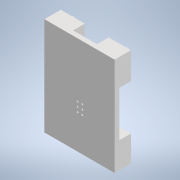
# Autodesk Inventor part: Soldering_Jig_Swerve
Saved by Autodesk Inventor 2022 (Build 260153000, 153)
## iProperties
Created: 2024-02-02
Part Number: Soldering_Jig_Swerve
Material: Generic
Document SubType Name: Modeling
Designer: Paul
Density: 1 g/cm^3
Appearance: Default
Author: Paul
Autodesk Inventor part; units mm, degrees
ref_plane "YZ Plane" through (0, 0, 0) normal (1, 0, 0) x (0, 1, 0)
ref_plane "XZ Plane" through (0, 0, 0) normal (0, 1, 0) x (-1, 0, 0)
ref_plane "XY Plane" through (0, 0, 0) normal (0, 0, 1) x (1, 0, 0)
sketch "Sketch1" plane through (0, 0, 0) normal (0, 0, 1) x (1, 0, 0)
  line L0 (-22.948, 8.421) -> (-22.948, -44.919) projected
  line L1 (-22.948, -44.919) -> (15.152, -44.919) projected
  line L2 (15.152, -44.919) -> (15.152, 8.421) projected
  line L3 (15.152, 8.421) -> (-22.948, 8.421) projected
  circle A0 centre (10.834, 4.103) radius 2.286 projected
  circle A1 centre (-18.63, 4.103) radius 2.286 projected
  circle A2 centre (-18.63, -40.601) radius 2.286 projected
  circle A3 centre (10.834, -40.601) radius 2.286 projected
  point P0 (0, 0)
extrude "Extrusion1" add sketch "Sketch1" along normal blind 2.54 contours L3 L2 L1 L0 | A0 | A1 | A2 | A3
sketch "Sketch2" plane through (0, 0, 0) normal (0, 0, -1) x (-1, 0, 0)
  line L0 (22.948, 8.421) -> (22.948, -44.919) projected
  line L1 (10.492, -0.541) -> (22.948, -0.541)
  line L2 (22.948, -0.541) -> (22.948, -18.939)
  line L3 (22.948, -18.939) -> (10.492, -18.939)
  line L4 (10.492, -18.939) -> (10.492, -0.541)
  line L5 (22.948, -22.163) -> (10.492, -22.163)
  line L6 (10.492, -22.163) -> (10.492, -35.163)
  line L7 (10.492, -35.163) -> (22.948, -35.163)
  line L8 (22.948, -35.163) -> (22.948, -22.163)
  line L9 (22.948, -44.919) -> (-15.152, -44.919) projected
  line L10 (8.874, -44.919) -> (-4.126, -44.919)
  line L11 (-4.126, -44.919) -> (-4.126, -32.448)
  line L12 (-4.126, -32.448) -> (8.874, -32.448)
  line L13 (8.874, -32.448) -> (8.874, -44.919)
  line L14 (-15.152, -44.919) -> (-15.152, 8.421) projected
  line L15 (-15.152, -30.845) -> (-2.427, -30.845)
  line L16 (-2.427, -30.845) -> (-2.427, -6.129)
  line L17 (-2.427, -6.129) -> (-15.152, -6.129)
  line L18 (-15.152, -6.129) -> (-15.152, -30.845)
  line L19 (-15.152, 8.421) -> (22.948, 8.421) projected
  line L20 (9.89, 8.421) -> (-3.11, 8.421)
  line L21 (-3.11, 8.421) -> (-3.11, -4.05)
  line L22 (-3.11, -4.05) -> (9.89, -4.05)
  line L23 (9.89, -4.05) -> (9.89, 8.421)
  line L24 (8.374, -32.948) -> (8.374, -44.198) projected
  line L25 (-3.626, -44.198) -> (-3.626, -32.948) projected
  line L26 (-1.876, -32.948) -> (-3.426, -32.948) projected
  line L27 (-2.927, -30.145) -> (-2.927, -28.595) projected
  line L28 (-2.927, -30.345) -> (-14.177, -30.345) projected
  line L29 (-2.927, -14.629) -> (-14.177, -14.629) projected
  line L30 (-14.177, -18.345) -> (-2.927, -18.345) projected
  line L31 (-14.177, -6.629) -> (-2.927, -6.629) projected
  line L32 (-2.41, -3.55) -> (-0.86, -3.55) projected
  line L33 (-2.61, -3.55) -> (-2.61, 7.7) projected
  line L34 (9.39, 7.7) -> (9.39, -3.55) projected
  line L35 (10.992, -1.041) -> (22.242, -1.041) projected
  line L36 (10.992, -1.241) -> (10.992, -2.791) projected
  line L37 (22.242, -9.041) -> (10.992, -9.041) projected
  line L38 (10.992, -10.439) -> (22.242, -10.439) projected
  line L39 (10.992, -10.639) -> (10.992, -12.189) projected
  line L40 (22.242, -18.439) -> (10.992, -18.439) projected
  line L41 (10.992, -22.663) -> (22.242, -22.663) projected
  line L42 (22.242, -34.663) -> (10.992, -34.663) projected
  line L43 (10.992, -32.913) -> (10.992, -34.463) projected
  point P0 (0, 0)
  dimension "d2" = 0.5
  dimension "d3" = 0.5
  dimension "d4" = 0.5
  dimension "d5" = 0.5
  dimension "d6" = 0.5
  dimension "d7" = 0.5
  dimension "d8" = 0.5
  dimension "d9" = 0.5
  dimension "d10" = 0.5
  dimension "d11" = 0.5
  dimension "d12" = 0.5
  dimension "d13" = 0.5
  dimension "d14" = 0.5
  dimension "d15" = 0.5
  constraints: 40 end point, 10 parallel, 6 point on line, 5 horizontal, 5 perpendicular
  measures "d2" distance between parallel lines of L6 L43
  measures "d3" distance between parallel lines of L42 L7
  measures "d4" distance between parallel lines of L5 L41
  measures "d5" distance between parallel lines of L40 L3
  measures "d6" distance between parallel lines of L1 L35
  measures "d7" distance between parallel lines of L34 L23
  measures "d8" distance between parallel lines of L22 L32
  measures "d9" distance between parallel lines of L21 L33
  measures "d10" distance between parallel lines of L17 L31
  measures "d11" distance between parallel lines of L16 L27
  measures "d12" distance between parallel lines of L28 L15
  measures "d13" distance between parallel lines of L25 L11
  measures "d14" distance between parallel lines of L12 L26
  measures "d15" distance between parallel lines of L13 L24
extrude "Extrusion2" add sketch "Sketch2" along normal blind 6.35 contours L0 L1 L4 L3 L5 L6 L7 L9 L13 L12 L11 L14 L15 L16 L17 L19 L21 L22 L23
sketch "Sketch3" plane through (0, 0, -6.35) normal (0, 0, -1) x (-1, 0, 0)
  line L0 (9.89, -4.05) -> (-3.11, -4.05) projected
  line L1 (10.492, -18.939) -> (10.492, -0.541) projected
  line L2 (10.492, -35.163) -> (10.492, -22.163) projected
  line L3 (-4.126, -32.448) -> (8.874, -32.448) projected
  line L4 (-2.427, -6.129) -> (-2.427, -30.845) projected
  line L5 (10.492, -4.05) -> (-2.427, -4.05)
  line L6 (-2.427, -4.05) -> (-2.427, -32.448)
  line L7 (-2.427, -32.448) -> (10.492, -32.448)
  line L8 (10.492, -32.448) -> (10.492, -4.05)
  line L9 (-1.411, -5.066) -> (9.476, -5.066)
  line L10 (9.476, -5.066) -> (9.476, -31.432)
  line L11 (9.476, -31.432) -> (-1.411, -31.432)
  line L12 (-1.411, -31.432) -> (-1.411, -5.066)
  point P0 (0, 0)
  dimension "d18" = 28.398
  dimension "d19" = 12.919
  dimension "d20" = 1.016
  constraints: 16 end point, 4 parallel, 2 perpendicular, 2 point on line, 1 horizontal, 3 other
  measures "d18" distance between parallel lines of L5 L7
  measures "d19" distance between parallel lines of L6 L8
  measures "d20" distance between parallel lines of L5 L9
extrude "Extrusion3" cut sketch "Sketch3" against normal blind 6.35 contours L9 L10 L11 L12
ref_plane "Work Plane1" through (-6.159, -27.632, -4.16) normal (0, 0, 1) x (1, 0, 0)
sketch "Sketch4" plane through (0, 0, 0) normal (0, 0, -1) x (-1, 0, 0)
  line L0 (6.159, -27.632) -> (6.159, -20.012) construction
  line L1 (1.119, -20.012) -> (1.119, -27.632) construction
  line L2 (6.159, -20.012) -> (1.119, -20.012) construction
  line L3 (1.119, -20.012) -> (1.119, -27.632) construction
  line L4 (1.119, -27.632) -> (6.159, -27.632) construction
  line L5 (6.159, -27.632) -> (6.159, -20.012) construction
  line L6 (0.611, -19.504) -> (6.667, -19.504)
  line L7 (6.667, -19.504) -> (6.667, -28.14)
  line L8 (6.667, -28.14) -> (0.611, -28.14)
  line L9 (0.611, -28.14) -> (0.611, -19.504)
  point P0 (0, 0)
  dimension "d23" = 0.508
  constraints: 16 end point, 4 parallel, 2 perpendicular, 1 horizontal, 3 other
  measures "d23" distance between parallel lines of L0 L7
extrude "Extrusion4" add sketch "Sketch4" along normal up to surface (4.16 mm away)
sketch "Sketch5" plane through (-0.611, -28.14, -4.16) normal (0, 0, -1) x (-1, 0, 0)
  circle A0 centre (4.298, 6.858) radius 0.5 projected
  circle A1 centre (4.298, 4.318) radius 0.5 projected
  circle A2 centre (4.298, 1.778) radius 0.5 projected
  circle A3 centre (1.758, 1.778) radius 0.5 projected
  circle A4 centre (1.758, 4.318) radius 0.5 projected
  circle A5 centre (1.758, 6.858) radius 0.5 projected
  point P0 (-0.611, 28.14)
extrude "Extrusion5" cut sketch "Sketch5" against normal through all
sketch "Sketch6" plane through (0, 0, -6.35) normal (0, 0, -1) x (-1, 0, 0)
  circle A0 centre (18.63, 4.103) radius 2.286 projected
  circle A1 centre (18.63, -40.601) radius 2.286 projected
  circle A2 centre (-10.834, -40.601) radius 2.286 projected
  circle A3 centre (-10.834, 4.103) radius 2.286 projected
  circle A4 centre (18.63, 4.103) radius 2.0955
  circle A5 centre (18.63, -40.601) radius 2.0955
  circle A6 centre (-10.834, -40.601) radius 2.0955
  circle A7 centre (-10.834, 4.103) radius 2.0955
  point P0 (0, 0)
  dimension "d28" = 4.191
  constraints: 4 centre point, 3 equal radius
  measures "d28" diameter of A4
extrude "Extrusion6" add sketch "Sketch6" along normal blind 2.54 contours A4 | A5 | A6 | A7
equation "\"d3\" = d2"
equation "\"d4\" = d2"
equation "\"d5\" = d2"
equation "\"d6\" = d2"
equation "\"d7\" = d2"
equation "\"d8\" = d2"
equation "\"d9\" = d2"
equation "\"d10\" = d2"
equation "\"d11\" = d2"
equation "\"d12\" = d2"
equation "\"d13\" = d2"
equation "\"d14\" = d2"
equation "\"d15\" = d2"
body "Solid1"
